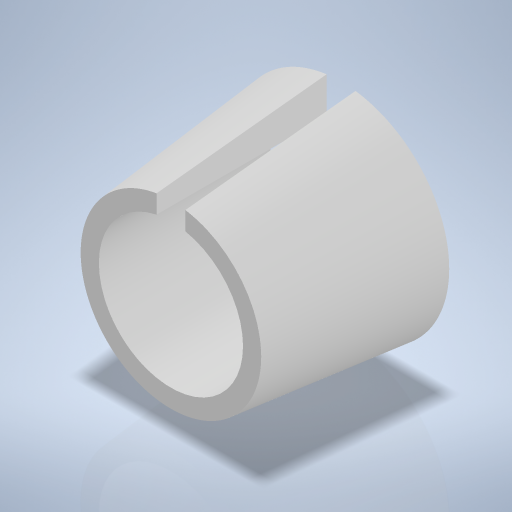
# Autodesk Inventor part: konus
Saved by Autodesk Inventor 2024 (Build 280153000, 153)
## iProperties
Created: 2024-04-30
Part Number: konus
Material: Generisch
Document SubType Name: Modeling
Designer: ffogue
Density: 1 g/cm^3
Appearance: Vorgabe
Author: ffogue
Autodesk Inventor part; units mm, degrees
note: some values were not read from the file. Chosen so that the rebuilt part matches the saved one: direction of "Bohrung1".
ref_plane "YZ Plane" through (0, 0, 0) normal (1, 0, 0) x (0, 1, 0)
ref_plane "XZ Plane" through (0, 0, 0) normal (0, 1, 0) x (-1, 0, 0)
ref_plane "XY Plane" through (0, 0, 0) normal (0, 0, 1) x (1, 0, 0)
sketch "Skizze1" plane through (0, 0, 0) normal (0, 1, 0) x (-1, 0, 0)
  circle A0 centre (0, 0) radius 7.5
  dimension "d0" = 15
  constraints: 1 centre point, 1 coincident
  measures "d0" diameter of A0
extrude "Extrusion1" add sketch "Skizze1" against normal blind 11.8
draft "Flächenverjüngung1" angle 6 pull direction (0, -1, 0) faces at (-7.4757, -7.8667, -0.6035) fixed edges at (7.5, 0, 0)
sketch "Skizze2" plane through (0, 0, 0) normal (0, 1, 0) x (1, 0, 0)
  circle A0 centre (0, 0) radius 7.5 projected
  constraints: 1 coincident
hole "Bohrung1" at (0, 0, 0) direction (0, -1, 0) diameter 10 depth 11.8
sketch "Skizze4" plane through (0, 0, 0) normal (0, 1, 0) x (1, 0, 0)
  line L0 (1, -7.5) -> (-1, -7.5)
  line L1 (-1, -7.5) -> (-1, -4.899)
  line L2 (1, -4.899) -> (1, -7.5)
  circle A0 centre (0, 0) radius 5 projected
  circle A1 centre (0, 0) radius 7.5 projected
  point P0 (0, -7.5)
  point P1 (-1, -7.433)
  point P2 (1, -7.433)
  point P3 (0, -7.5)
  dimension "d12" = 2
  constraints: 6 end point, 2 point on circle, 1 horizontal, 1 midpoint, 1 parallel, 1 perpendicular, 1 tangent, 1 vertical alignment
  measures "d12" distance between parallel lines of L1 L2
extrude "Extrusion2" cut sketch "Skizze4" against normal up to surface (11.8 mm away) contours A1 L1 A0 L2 picked at (0, -5.8258)
